Autodesk Inventor part; units mm, degrees
(part 5 of 6)
  arc A2268 (-444.6554, 18.0951) -> (-444.477, 18.6759) centre (-445.0102, 18.5219) ccw
  arc A2269 (-444.477, 18.6759) -> (-444.8927, 19.0646) centre (-445.0103, 18.5222) ccw
  arc A2270 (-444.8927, 19.0646) -> (-445.2136, 19.0814) centre (-445.1047, 18.0874) ccw
  arc A2271 (-445.3689, 19.174) -> (-445.2136, 19.0814) centre (-445.23, 19.2305) ccw
  arc A2272 (-445.5028, 19.7209) -> (-445.3689, 19.174) centre (-421.46, 25.315) ccw
  arc A2273 (-445.4078, 19.8747) -> (-445.5028, 19.7209) centre (-445.3534, 19.7349) ccw
  arc A2274 (-445.4078, 19.8747) -> (-445.1309, 20.0378) centre (-445.7702, 20.8067) ccw
  arc A2275 (-445.1309, 20.0378) -> (-444.9417, 20.5746) centre (-445.4857, 20.4646) ccw
  arc A2276 (-444.9417, 20.5746) -> (-445.3681, 21.0073) centre (-445.4858, 20.4649) ccw
  arc A2277 (-445.3681, 21.0073) -> (-445.6891, 21.0241) centre (-445.5801, 20.03) ccw
  arc A2278 (-445.7718, 21.0387) -> (-445.6891, 21.0241) centre (-445.7054, 21.1732) ccw
  arc A2279 (-445.8827, 21.7261) -> (-445.7718, 21.0387) centre (-421.46, 25.315) ccw
  arc A2280 (-445.8088, 21.7659) -> (-445.8827, 21.7261) centre (-445.7774, 21.6192) ccw
  arc A2281 (-445.8088, 21.7659) -> (-445.5094, 21.8828) centre (-446.0181, 22.7438) ccw
  arc A2282 (-445.5094, 21.8828) -> (-445.2408, 22.4277) centre (-445.7917, 22.3606) ccw
  arc A2283 (-445.2408, 22.4277) -> (-445.5892, 22.8777) centre (-445.7917, 22.361) ccw
  arc A2284 (-445.5892, 22.8777) -> (-445.9034, 22.9454) centre (-445.9542, 21.9467) ccw
  arc A2285 (-446.0419, 23.0615) -> (-445.9034, 22.9454) centre (-445.8958, 23.0952) ccw
  arc A2286 (-446.0869, 23.6228) -> (-446.0419, 23.0615) centre (-421.46, 25.315) ccw
  arc A2287 (-445.9687, 23.7595) -> (-446.0869, 23.6228) centre (-445.9373, 23.6128) ccw
  arc A2288 (-445.9687, 23.7595) -> (-445.6693, 23.8764) centre (-446.1779, 24.7374) ccw
  arc A2289 (-445.6693, 23.8764) -> (-445.397, 24.3762) centre (-445.9516, 24.3542) ccw
  arc A2290 (-445.397, 24.3762) -> (-445.749, 24.8713) centre (-445.9516, 24.3546) ccw
  arc A2291 (-445.749, 24.8713) -> (-446.0632, 24.939) centre (-446.114, 23.9403) ccw
  arc A2292 (-446.1425, 24.9666) -> (-446.0632, 24.939) centre (-446.0556, 25.0888) ccw
  arc A2293 (-446.1425, 25.6629) -> (-446.1425, 24.9666) centre (-421.46, 25.315) ccw
  arc A2294 (-446.0632, 25.6905) -> (-446.1425, 25.6629) centre (-446.0556, 25.5406) ccw
  arc A2295 (-446.0632, 25.6905) -> (-445.749, 25.7581) centre (-446.114, 26.6892) ccw
  arc A2296 (-445.749, 25.7581) -> (-445.397, 26.2533) centre (-445.9516, 26.2749) ccw
  arc A2297 (-445.397, 26.2533) -> (-445.6693, 26.7531) centre (-445.9516, 26.2752) ccw
  arc A2298 (-445.6693, 26.7531) -> (-445.9687, 26.8699) centre (-446.1779, 25.8921) ccw
  arc A2299 (-446.087, 27.0066) -> (-445.9687, 26.8699) centre (-445.9373, 27.0166) ccw
  arc A2300 (-446.042, 27.5679) -> (-446.087, 27.0066) centre (-421.46, 25.315) ccw
  arc A2301 (-445.9034, 27.6841) -> (-446.042, 27.5679) centre (-445.8958, 27.5343) ccw
  arc A2302 (-445.9034, 27.6841) -> (-445.5892, 27.7518) centre (-445.9542, 28.6828) ccw
  arc A2303 (-445.5892, 27.7518) -> (-445.2408, 28.2018) centre (-445.7918, 28.2685) ccw
  arc A2304 (-445.2408, 28.2018) -> (-445.5095, 28.7467) centre (-445.7918, 28.2688) ccw
  arc A2305 (-445.5095, 28.7467) -> (-445.8089, 28.8635) centre (-446.0181, 27.8857) ccw
  arc A2306 (-445.8828, 28.9034) -> (-445.8089, 28.8635) centre (-445.7775, 29.0102) ccw
  arc A2307 (-445.7719, 29.5908) -> (-445.8828, 28.9034) centre (-421.46, 25.315) ccw
  arc A2308 (-445.6892, 29.6054) -> (-445.7719, 29.5908) centre (-445.7055, 29.4563) ccw
  arc A2309 (-445.6892, 29.6054) -> (-445.3682, 29.6222) centre (-445.5802, 30.5994) ccw
  arc A2310 (-445.3682, 29.6222) -> (-444.9418, 30.0549) centre (-445.4859, 30.1646) ccw
  arc A2311 (-444.9418, 30.0549) -> (-445.131, 30.5917) centre (-445.4858, 30.1649) ccw
  arc A2312 (-445.131, 30.5917) -> (-445.4079, 30.7548) centre (-445.7703, 29.8227) ccw
  arc A2313 (-445.5029, 30.9086) -> (-445.4079, 30.7548) centre (-445.3536, 30.8946) ccw
  arc A2314 (-445.3691, 31.4555) -> (-445.5029, 30.9086) centre (-421.46, 25.315) ccw
  arc A2315 (-445.2138, 31.5481) -> (-445.3691, 31.4555) centre (-445.2301, 31.399) ccw
  arc A2316 (-445.2138, 31.5481) -> (-444.8928, 31.5649) centre (-445.1048, 32.5421) ccw
  arc A2317 (-444.8928, 31.5649) -> (-444.4772, 31.9536) centre (-445.0105, 32.1072) ccw
  arc A2318 (-444.4772, 31.9536) -> (-444.6556, 32.5344) centre (-445.0104, 32.1076) ccw
  arc A2319 (-444.6556, 32.5344) -> (-444.9325, 32.6974) centre (-445.2949, 31.7654) ccw
  arc A2320 (-444.9991, 32.7486) -> (-444.9325, 32.6974) centre (-444.8782, 32.8372) ccw
  arc A2321 (-444.7801, 33.4095) -> (-444.9991, 32.7486) centre (-421.46, 25.315) ccw
  arc A2322 (-444.6961, 33.4107) -> (-444.7801, 33.4095) centre (-444.736, 33.2661) ccw
  arc A2323 (-444.6961, 33.4107) -> (-444.3766, 33.3762) centre (-444.4302, 34.3747) ccw
  arc A2324 (-444.3766, 33.3762) -> (-443.8867, 33.7355) centre (-444.4064, 33.9304) ccw
  arc A2325 (-443.8867, 33.7355) -> (-443.988, 34.2955) centre (-444.4062, 33.9307) ccw
  arc A2326 (-443.988, 34.2955) -> (-444.2354, 34.5006) centre (-444.7416, 33.6382) ccw
  arc A2327 (-444.3047, 34.6676) -> (-444.2354, 34.5006) centre (-444.1594, 34.63) ccw
  arc A2328 (-444.0854, 35.1862) -> (-444.3047, 34.6676) centre (-421.46, 25.315) ccw
  arc A2329 (-443.9173, 35.2529) -> (-444.0854, 35.1862) centre (-443.9572, 35.1083) ccw
  arc A2330 (-443.9173, 35.2529) -> (-443.5978, 35.2183) centre (-443.6514, 36.2169) ccw
  arc A2331 (-443.5978, 35.2183) -> (-443.1255, 35.5359) centre (-443.6276, 35.7725) ccw
  arc A2332 (-443.1255, 35.5359) -> (-443.2091, 36.1376) centre (-443.6274, 35.7728) ccw
  arc A2333 (-443.2091, 36.1376) -> (-443.4566, 36.3427) centre (-443.9628, 35.4803) ccw
  arc A2334 (-443.5142, 36.4038) -> (-443.4566, 36.3427) centre (-443.3806, 36.4721) ccw
  arc A2335 (-443.1927, 37.0214) -> (-443.5142, 36.4038) centre (-421.46, 25.315) ccw
  arc A2336 (-443.1096, 37.0093) -> (-443.1927, 37.0214) centre (-443.172, 36.8729) ccw
  arc A2337 (-443.1096, 37.0093) -> (-442.7996, 36.9242) centre (-442.6934, 37.9186) ccw
  arc A2338 (-442.7996, 36.9242) -> (-442.2587, 37.2009) centre (-442.7407, 37.4761) ccw
  arc A2339 (-442.2587, 37.2009) -> (-442.2695, 37.7699) centre (-442.7405, 37.4764) ccw
  arc A2340 (-442.2695, 37.7699) -> (-442.481, 38.0118) centre (-443.1182, 37.2411) ccw
  arc A2341 (-442.5228, 38.1877) -> (-442.481, 38.0118) centre (-442.3855, 38.1274) ccw
  arc A2342 (-442.2237, 38.6648) -> (-442.5228, 38.1877) centre (-421.46, 25.315) ccw
  arc A2343 (-442.0472, 38.7038) -> (-442.2237, 38.6648) centre (-442.1096, 38.5674) ccw
  arc A2344 (-442.0472, 38.7038) -> (-441.7373, 38.6188) centre (-441.6311, 39.6131) ccw
  arc A2345 (-441.7373, 38.6188) -> (-441.2204, 38.857) centre (-441.6783, 39.1706) ccw
  arc A2346 (-441.2204, 38.857) -> (-441.2071, 39.4644) centre (-441.6781, 39.1709) ccw
  arc A2347 (-441.2071, 39.4644) -> (-441.4187, 39.7063) centre (-442.0558, 38.9356) ccw
  arc A2348 (-441.4658, 39.7758) -> (-441.4187, 39.7063) centre (-441.3231, 39.822) ccw
  arc A2349 (-441.05, 40.3343) -> (-441.4658, 39.7758) centre (-421.46, 25.315) ccw
  arc A2350 (-440.9699, 40.3091) -> (-441.05, 40.3343) centre (-441.0533, 40.1844) ccw
  arc A2351 (-440.9699, 40.3091) -> (-440.6775, 40.1757) centre (-440.4142, 41.1405) ccw
  arc A2352 (-440.6775, 40.1757) -> (-440.0994, 40.3627) centre (-440.5314, 40.7112) ccw
  arc A2353 (-440.0994, 40.3627) -> (-440.0194, 40.9262) centre (-440.5312, 40.7115) ccw
  arc A2354 (-440.0194, 40.9262) -> (-440.1897, 41.1987) centre (-440.9415, 40.5393) ccw
  arc A2355 (-440.2029, 41.379) -> (-440.1897, 41.1987) centre (-440.0769, 41.2976) ccw
  arc A2356 (-439.8317, 41.8023) -> (-440.2029, 41.379) centre (-421.46, 25.315) ccw
  arc A2357 (-439.6512, 41.8127) -> (-439.8317, 41.8023) centre (-439.7345, 41.688) ccw
  arc A2358 (-439.6512, 41.8127) -> (-439.3587, 41.6794) centre (-439.0955, 42.6441) ccw
  arc A2359 (-439.3587, 41.6794) -> (-438.8105, 41.8323) centre (-439.2126, 42.2148) ccw
  arc A2360 (-438.8105, 41.8323) -> (-438.7006, 42.4298) centre (-439.2124, 42.2151) ccw
  arc A2361 (-438.7006, 42.4298) -> (-438.8709, 42.7023) centre (-439.6228, 42.0429) ccw
  arc A2362 (-438.9064, 42.7784) -> (-438.8709, 42.7023) centre (-438.7582, 42.8012) ccw
  arc A2363 (-438.4069, 43.2635) -> (-438.9064, 42.7784) centre (-421.46, 25.315) ccw
  arc A2364 (-438.3319, 43.2258) -> (-438.4069, 43.2635) centre (-438.4341, 43.116) ccw
  arc A2365 (-438.3319, 43.2258) -> (-438.0644, 43.0476) centre (-437.6509, 43.9581) ccw
  arc A2366 (-438.0644, 43.0476) -> (-437.464, 43.1401) centre (-437.8349, 43.5529) ccw
  arc A2367 (-437.464, 43.1401) -> (-437.2952, 43.6836) centre (-437.8346, 43.5532) ccw
  arc A2368 (-437.2952, 43.6836) -> (-437.4199, 43.9798) centre (-438.2672, 43.4486) ccw
  arc A2369 (-437.4043, 44.1599) -> (-437.4199, 43.9798) centre (-437.2928, 44.0595) ccw
  arc A2370 (-436.9703, 44.5187) -> (-437.4043, 44.1599) centre (-421.46, 25.315) ccw
  arc A2371 (-436.7904, 44.5002) -> (-436.9703, 44.5187) centre (-436.8926, 44.3903) ccw
  arc A2372 (-436.7904, 44.5002) -> (-436.523, 44.322) centre (-436.1094, 45.2324) ccw
  arc A2373 (-436.523, 44.322) -> (-435.9574, 44.3856) centre (-436.2935, 44.8273) ccw
  arc A2374 (-435.9574, 44.3856) -> (-435.7537, 44.9579) centre (-436.2932, 44.8275) ccw
  arc A2375 (-435.7537, 44.9579) -> (-435.8784, 45.2541) centre (-436.7257, 44.7229) ccw
  arc A2376 (-435.9014, 45.3349) -> (-435.8784, 45.2541) centre (-435.7514, 45.3338) ccw
  arc A2377 (-435.331, 45.7342) -> (-435.9014, 45.3349) centre (-421.46, 25.315) ccw
  arc A2378 (-435.2629, 45.6851) -> (-435.331, 45.7342) centre (-435.3812, 45.5929) ccw
  arc A2379 (-435.2629, 45.6851) -> (-435.0272, 45.4665) centre (-434.4739, 46.2995) ccw
  arc A2380 (-435.0272, 45.4665) -> (-434.4197, 45.4621) centre (-434.7201, 45.9288) ccw
  arc A2381 (-434.4197, 45.4621) -> (-434.1665, 45.9718) centre (-434.7198, 45.929) ccw
  arc A2382 (-434.1665, 45.9718) -> (-434.2424, 46.2841) centre (-435.1635, 45.8947) ccw
  arc A2383 (-434.1983, 46.4594) -> (-434.2424, 46.2841) centre (-434.1043, 46.3425) ccw
  arc A2384 (-433.7127, 46.7445) -> (-434.1983, 46.4594) centre (-421.46, 25.315) ccw
  arc A2385 (-433.5381, 46.6976) -> (-433.7127, 46.7445) centre (-433.6564, 46.6054) ccw
  arc A2386 (-433.5381, 46.6976) -> (-433.3024, 46.479) centre (-432.7491, 47.3119) ccw
  arc A2387 (-433.3024, 46.479) -> (-432.734, 46.4517) centre (-432.9953, 46.9413) ccw
  arc A2388 (-432.734, 46.4517) -> (-432.4417, 46.9843) centre (-432.995, 46.9415) ccw
  arc A2389 (-432.4417, 46.9843) -> (-432.5176, 47.2965) centre (-433.4387, 46.9071) ccw
  arc A2390 (-432.5274, 47.38) -> (-432.5176, 47.2965) centre (-432.3795, 47.355) ccw
  arc A2391 (-431.9006, 47.6833) -> (-432.5274, 47.38) centre (-421.46, 25.315) ccw
  arc A2392 (-431.8412, 47.6239) -> (-431.9006, 47.6833) centre (-431.9728, 47.5518) ccw
  arc A2393 (-431.8412, 47.6239) -> (-431.6434, 47.3706) centre (-430.9644, 48.1048) ccw
  arc A2394 (-431.6434, 47.3706) -> (-431.0444, 47.2695) centre (-431.2666, 47.7781) ccw
  arc A2395 (-431.0444, 47.2695) -> (-430.7132, 47.7323) centre (-431.2663, 47.7782) ccw
  arc A2396 (-430.7132, 47.7323) -> (-430.7384, 48.0527) centre (-431.7097, 47.815) ccw
  arc A2397 (-430.6669, 48.2188) -> (-430.7384, 48.0527) centre (-430.5927, 48.0884) ccw
  arc A2398 (-430.1421, 48.4228) -> (-430.6669, 48.2188) centre (-421.46, 25.315) ccw
  arc A2399 (-429.9772, 48.3487) -> (-430.1421, 48.4228) centre (-430.1087, 48.2766) ccw
  arc A2400 (-429.9772, 48.3487) -> (-429.7794, 48.0954) centre (-429.1004, 48.8295) ccw
  arc A2401 (-429.7794, 48.0954) -> (-429.2225, 47.9779) centre (-429.4025, 48.5028) ccw
  arc A2402 (-429.2225, 47.9779) -> (-428.8491, 48.4571) centre (-429.4022, 48.503) ccw
  arc A2403 (-428.8491, 48.4571) -> (-428.8743, 48.7775) centre (-429.8457, 48.5398) ccw
  arc A2404 (-428.8707, 48.8614) -> (-428.8743, 48.7775) centre (-428.7286, 48.8131) ccw
  arc A2405 (-428.2036, 49.061) -> (-428.8707, 48.8614) centre (-421.46, 25.315) ccw
  arc A2406 (-428.1544, 48.9929) -> (-428.2036, 49.061) centre (-428.2958, 48.9427) ccw
  arc A2407 (-428.1544, 48.9929) -> (-427.9995, 48.7113) centre (-427.2122, 49.3279) ccw
  arc A2408 (-427.9995, 48.7113) -> (-427.4242, 48.5161) centre (-427.5626, 49.0536) ccw
  arc A2409 (-427.4242, 48.5161) -> (-427.0235, 48.9202) centre (-427.5622, 49.0536) ccw
  arc A2410 (-427.0235, 48.9202) -> (-426.9974, 49.2405) centre (-427.9942, 49.1606) ccw
  arc A2411 (-426.9003, 49.393) -> (-426.9974, 49.2405) centre (-426.8478, 49.2525) ccw
  arc A2412 (-426.3497, 49.5109) -> (-426.9003, 49.393) centre (-421.46, 25.315) ccw
  arc A2413 (-426.1987, 49.4114) -> (-426.3497, 49.5109) centre (-426.34, 49.3612) ccw
  arc A2414 (-426.1987, 49.4114) -> (-426.0438, 49.1299) centre (-425.2565, 49.7465) ccw
  arc A2415 (-426.0438, 49.1299) -> (-425.5128, 48.9251) centre (-425.6068, 49.4721) ccw
  arc A2416 (-425.5128, 48.9251) -> (-425.0678, 49.3387) centre (-425.6065, 49.4721) ccw
  arc A2417 (-425.0678, 49.3387) -> (-425.0416, 49.659) centre (-426.0384, 49.5791) ccw
  arc A2418 (-425.0246, 49.7413) -> (-425.0416, 49.659) centre (-424.8921, 49.671) ccw
  arc A2419 (-424.3343, 49.8321) -> (-425.0246, 49.7413) centre (-421.46, 25.315) ccw
  arc A2420 (-424.2966, 49.757) -> (-424.3343, 49.8321) centre (-424.4441, 49.7299) ccw
  arc A2421 (-424.2966, 49.757) -> (-424.1885, 49.4544) centre (-423.313, 49.9377) ccw
  arc A2422 (-424.1885, 49.4544) -> (-423.6517, 49.1699) centre (-423.7026, 49.7226) ccw
  arc A2423 (-423.6517, 49.1699) -> (-423.1917, 49.5051) centre (-423.7023, 49.7226) ccw
  arc A2424 (-423.1917, 49.5051) -> (-423.1149, 49.8171) centre (-424.1117, 49.8971) ccw
  arc A2425 (-422.9947, 49.9522) -> (-423.1149, 49.8171) centre (-422.9653, 49.8052) ccw
  arc A2426 (-422.4324, 49.9808) -> (-422.9947, 49.9522) centre (-421.46, 25.315) ccw
  arc A2427 (-422.2992, 49.8586) -> (-422.4324, 49.9808) centre (-422.4467, 49.8315) ccw
  arc A2428 (-422.2992, 49.8586) -> (-422.1911, 49.556) centre (-421.3156, 50.0392) ccw
  arc A2429 (-422.1911, 49.556) -> (-421.6995, 49.2692) centre (-421.7052, 49.8242) ccw
  arc A2430 (-421.6995, 49.2692) -> (-421.1943, 49.6066) centre (-421.7048, 49.8242) ccw
  arc A2431 (-421.1943, 49.6066) -> (-421.1174, 49.9187) centre (-422.1142, 49.9986) ccw
  arc A2432 (-421.0854, 50) -> (-421.1174, 49.9187) centre (-420.9679, 49.9067) ccw
  line L316 (-421.0854, 50) -> (-420.4705, 50)
  arc A2433 (-420.3218, 49.8696) -> (-420.4705, 50) centre (-420.4705, 49.85) ccw
  arc A2434 (-420.3218, 49.8696) -> (-420.2292, 49.5618) centre (-419.3304, 50) ccw
  arc A2435 (-420.2292, 49.5618) -> (-419.7302, 49.25) centre (-419.7304, 49.805) ccw
  arc A2436 (-419.7302, 49.25) -> (-419.2311, 49.5618) centre (-419.73, 49.805) ccw
  arc A2437 (-419.2311, 49.5618) -> (-419.1385, 49.8696) centre (-420.13, 50) ccw
  arc A2438 (-418.9898, 50) -> (-419.1385, 49.8696) centre (-418.9898, 49.85) ccw
  line L317 (-418.9898, 50) -> (-418.4705, 50)
  arc A2439 (-418.3218, 49.8696) -> (-418.4705, 50) centre (-418.4705, 49.85) ccw
  arc A2440 (-418.3218, 49.8696) -> (-418.2292, 49.5618) centre (-417.3304, 50) ccw
  arc A2441 (-418.2292, 49.5618) -> (-417.7302, 49.25) centre (-417.7304, 49.805) ccw
  arc A2442 (-417.7302, 49.25) -> (-417.2311, 49.5618) centre (-417.73, 49.805) ccw
  arc A2443 (-417.2311, 49.5618) -> (-417.1385, 49.8696) centre (-418.13, 50) ccw
  arc A2444 (-416.9898, 50) -> (-417.1385, 49.8696) centre (-416.9898, 49.85) ccw
  line L318 (-416.9898, 50) -> (-416.4705, 50)
  arc A2445 (-416.3218, 49.8696) -> (-416.4705, 50) centre (-416.4705, 49.85) ccw
  arc A2446 (-416.3218, 49.8696) -> (-416.2292, 49.5618) centre (-415.3304, 50) ccw
  arc A2447 (-416.2292, 49.5618) -> (-415.7302, 49.25) centre (-415.7304, 49.805) ccw
  arc A2448 (-415.7302, 49.25) -> (-415.2311, 49.5618) centre (-415.73, 49.805) ccw
  arc A2449 (-415.2311, 49.5618) -> (-415.1385, 49.8696) centre (-416.13, 50) ccw
  arc A2450 (-414.9898, 50) -> (-415.1385, 49.8696) centre (-414.9898, 49.85) ccw
  line L319 (-414.9898, 50) -> (-414.4705, 50)
  arc A2451 (-414.3218, 49.8696) -> (-414.4705, 50) centre (-414.4705, 49.85) ccw
  arc A2452 (-414.3218, 49.8696) -> (-414.2292, 49.5618) centre (-413.3304, 50) ccw
  arc A2453 (-414.2292, 49.5618) -> (-413.7302, 49.25) centre (-413.7304, 49.805) ccw
  arc A2454 (-413.7302, 49.25) -> (-413.2311, 49.5618) centre (-413.73, 49.805) ccw
  arc A2455 (-413.2311, 49.5618) -> (-413.1385, 49.8696) centre (-414.13, 50) ccw
  arc A2456 (-412.9898, 50) -> (-413.1385, 49.8696) centre (-412.9898, 49.85) ccw
  line L320 (-412.9898, 50) -> (-412.4705, 50)
  arc A2457 (-412.3218, 49.8696) -> (-412.4705, 50) centre (-412.4705, 49.85) ccw
  arc A2458 (-412.3218, 49.8696) -> (-412.2292, 49.5618) centre (-411.3304, 50) ccw
  arc A2459 (-412.2292, 49.5618) -> (-411.7302, 49.25) centre (-411.7304, 49.805) ccw
  arc A2460 (-411.7302, 49.25) -> (-411.2311, 49.5618) centre (-411.73, 49.805) ccw
  arc A2461 (-411.2311, 49.5618) -> (-411.1385, 49.8696) centre (-412.13, 50) ccw
  arc A2462 (-410.9898, 50) -> (-411.1385, 49.8696) centre (-410.9898, 49.85) ccw
  line L321 (-410.9898, 50) -> (-410.4705, 50)
  arc A2463 (-410.3218, 49.8696) -> (-410.4705, 50) centre (-410.4705, 49.85) ccw
  arc A2464 (-410.3218, 49.8696) -> (-410.2292, 49.5618) centre (-409.3304, 50) ccw
  arc A2465 (-410.2292, 49.5618) -> (-409.7302, 49.25) centre (-409.7304, 49.805) ccw
  arc A2466 (-409.7302, 49.25) -> (-409.2311, 49.5618) centre (-409.73, 49.805) ccw
  arc A2467 (-409.2311, 49.5618) -> (-409.1385, 49.8696) centre (-410.13, 50) ccw
  arc A2468 (-408.9898, 50) -> (-409.1385, 49.8696) centre (-408.9898, 49.85) ccw
  line L322 (-408.9898, 50) -> (-408.4705, 50)
  arc A2469 (-408.3218, 49.8696) -> (-408.4705, 50) centre (-408.4705, 49.85) ccw
  arc A2470 (-408.3218, 49.8696) -> (-408.2292, 49.5618) centre (-407.3304, 50) ccw
  arc A2471 (-408.2292, 49.5618) -> (-407.7302, 49.25) centre (-407.7304, 49.805) ccw
  arc A2472 (-407.7302, 49.25) -> (-407.2311, 49.5618) centre (-407.73, 49.805) ccw
  arc A2473 (-407.2311, 49.5618) -> (-407.1385, 49.8696) centre (-408.13, 50) ccw
  arc A2474 (-406.9898, 50) -> (-407.1385, 49.8696) centre (-406.9898, 49.85) ccw
  line L323 (-406.9898, 50) -> (-406.4705, 50)
  arc A2475 (-406.3218, 49.8696) -> (-406.4705, 50) centre (-406.4705, 49.85) ccw
  arc A2476 (-406.3218, 49.8696) -> (-406.2292, 49.5618) centre (-405.3304, 50) ccw
  arc A2477 (-406.2292, 49.5618) -> (-405.7302, 49.25) centre (-405.7304, 49.805) ccw
  arc A2478 (-405.7302, 49.25) -> (-405.2311, 49.5618) centre (-405.73, 49.805) ccw
  arc A2479 (-405.2311, 49.5618) -> (-405.1385, 49.8696) centre (-406.13, 50) ccw
  arc A2480 (-404.9898, 50) -> (-405.1385, 49.8696) centre (-404.9898, 49.85) ccw
  line L324 (-404.9898, 50) -> (-404.4705, 50)
  arc A2481 (-404.3218, 49.8696) -> (-404.4705, 50) centre (-404.4705, 49.85) ccw
  arc A2482 (-404.3218, 49.8696) -> (-404.2292, 49.5618) centre (-403.3304, 50) ccw
  arc A2483 (-404.2292, 49.5618) -> (-403.7302, 49.25) centre (-403.7304, 49.805) ccw
  arc A2484 (-403.7302, 49.25) -> (-403.2311, 49.5618) centre (-403.73, 49.805) ccw
  arc A2485 (-403.2311, 49.5618) -> (-403.1385, 49.8696) centre (-404.13, 50) ccw
  arc A2486 (-402.9898, 50) -> (-403.1385, 49.8696) centre (-402.9898, 49.85) ccw
  line L325 (-402.9898, 50) -> (-402.4705, 50)
  arc A2487 (-402.3218, 49.8696) -> (-402.4705, 50) centre (-402.4705, 49.85) ccw
  arc A2488 (-402.3218, 49.8696) -> (-402.2292, 49.5618) centre (-401.3304, 50) ccw
  arc A2489 (-402.2292, 49.5618) -> (-401.7302, 49.25) centre (-401.7304, 49.805) ccw
  arc A2490 (-401.7302, 49.25) -> (-401.2311, 49.5618) centre (-401.73, 49.805) ccw
  arc A2491 (-401.2311, 49.5618) -> (-401.1385, 49.8696) centre (-402.13, 50) ccw
  arc A2492 (-400.9898, 50) -> (-401.1385, 49.8696) centre (-400.9898, 49.85) ccw
  line L326 (-400.9898, 50) -> (-400.4705, 50)
  arc A2493 (-400.3218, 49.8696) -> (-400.4705, 50) centre (-400.4705, 49.85) ccw
  arc A2494 (-400.3218, 49.8696) -> (-400.2292, 49.5618) centre (-399.3304, 50) ccw
  arc A2495 (-400.2292, 49.5618) -> (-399.7302, 49.25) centre (-399.7304, 49.805) ccw
  arc A2496 (-399.7302, 49.25) -> (-399.2311, 49.5618) centre (-399.73, 49.805) ccw
  arc A2497 (-399.2311, 49.5618) -> (-399.1385, 49.8696) centre (-400.13, 50) ccw
  arc A2498 (-398.9898, 50) -> (-399.1385, 49.8696) centre (-398.9898, 49.85) ccw
  line L327 (-398.9898, 50) -> (-398.4705, 50)
  arc A2499 (-398.3218, 49.8696) -> (-398.4705, 50) centre (-398.4705, 49.85) ccw
  arc A2500 (-398.3218, 49.8696) -> (-398.2292, 49.5618) centre (-397.3304, 50) ccw
  arc A2501 (-398.2292, 49.5618) -> (-397.7302, 49.25) centre (-397.7304, 49.805) ccw
  arc A2502 (-397.7302, 49.25) -> (-397.2311, 49.5618) centre (-397.73, 49.805) ccw
  arc A2503 (-397.2311, 49.5618) -> (-397.1385, 49.8696) centre (-398.13, 50) ccw
  arc A2504 (-396.9898, 50) -> (-397.1385, 49.8696) centre (-396.9898, 49.85) ccw
  line L328 (-396.9898, 50) -> (-396.4705, 50)
  arc A2505 (-396.3218, 49.8696) -> (-396.4705, 50) centre (-396.4705, 49.85) ccw
  arc A2506 (-396.3218, 49.8696) -> (-396.2292, 49.5618) centre (-395.3304, 50) ccw
  arc A2507 (-396.2292, 49.5618) -> (-395.7302, 49.25) centre (-395.7304, 49.805) ccw
  arc A2508 (-395.7302, 49.25) -> (-395.2311, 49.5618) centre (-395.73, 49.805) ccw
  arc A2509 (-395.2311, 49.5618) -> (-395.1385, 49.8696) centre (-396.13, 50) ccw
  arc A2510 (-394.9898, 50) -> (-395.1385, 49.8696) centre (-394.9898, 49.85) ccw
  line L329 (-394.9898, 50) -> (-394.4705, 50)
  arc A2511 (-394.3218, 49.8696) -> (-394.4705, 50) centre (-394.4705, 49.85) ccw
  arc A2512 (-394.3218, 49.8696) -> (-394.2292, 49.5618) centre (-393.3304, 50) ccw
  arc A2513 (-394.2292, 49.5618) -> (-393.7302, 49.25) centre (-393.7304, 49.805) ccw
  arc A2514 (-393.7302, 49.25) -> (-393.2311, 49.5618) centre (-393.73, 49.805) ccw
  arc A2515 (-393.2311, 49.5618) -> (-393.1385, 49.8696) centre (-394.13, 50) ccw
  arc A2516 (-392.9898, 50) -> (-393.1385, 49.8696) centre (-392.9898, 49.85) ccw
  line L330 (-392.9898, 50) -> (-392.4705, 50)
  arc A2517 (-392.3218, 49.8696) -> (-392.4705, 50) centre (-392.4705, 49.85) ccw
  arc A2518 (-392.3218, 49.8696) -> (-392.2292, 49.5618) centre (-391.3304, 50) ccw
  arc A2519 (-392.2292, 49.5618) -> (-391.7302, 49.25) centre (-391.7304, 49.805) ccw
  arc A2520 (-391.7302, 49.25) -> (-391.2311, 49.5618) centre (-391.73, 49.805) ccw
  arc A2521 (-391.2311, 49.5618) -> (-391.1385, 49.8696) centre (-392.13, 50) ccw
  arc A2522 (-390.9898, 50) -> (-391.1385, 49.8696) centre (-390.9898, 49.85) ccw
  line L331 (-390.9898, 50) -> (-390.4705, 50)
  arc A2523 (-390.3218, 49.8696) -> (-390.4705, 50) centre (-390.4705, 49.85) ccw
  arc A2524 (-390.3218, 49.8696) -> (-390.2292, 49.5618) centre (-389.3304, 50) ccw
  arc A2525 (-390.2292, 49.5618) -> (-389.7302, 49.25) centre (-389.7304, 49.805) ccw
  arc A2526 (-389.7302, 49.25) -> (-389.2311, 49.5618) centre (-389.73, 49.805) ccw
  arc A2527 (-389.2311, 49.5618) -> (-389.1385, 49.8696) centre (-390.13, 50) ccw
  arc A2528 (-388.9898, 50) -> (-389.1385, 49.8696) centre (-388.9898, 49.85) ccw
  line L332 (-388.9898, 50) -> (-388.4705, 50)
  arc A2529 (-388.3218, 49.8696) -> (-388.4705, 50) centre (-388.4705, 49.85) ccw
  arc A2530 (-388.3218, 49.8696) -> (-388.2292, 49.5618) centre (-387.3304, 50) ccw
  arc A2531 (-388.2292, 49.5618) -> (-387.7302, 49.25) centre (-387.7304, 49.805) ccw
  arc A2532 (-387.7302, 49.25) -> (-387.2311, 49.5618) centre (-387.73, 49.805) ccw
  arc A2533 (-387.2311, 49.5618) -> (-387.1385, 49.8696) centre (-388.13, 50) ccw
  arc A2534 (-386.9898, 50) -> (-387.1385, 49.8696) centre (-386.9898, 49.85) ccw
  line L333 (-386.9898, 50) -> (-386.4705, 50)
  arc A2535 (-386.3218, 49.8696) -> (-386.4705, 50) centre (-386.4705, 49.85) ccw
  arc A2536 (-386.3218, 49.8696) -> (-386.2292, 49.5618) centre (-385.3304, 50) ccw
  arc A2537 (-386.2292, 49.5618) -> (-385.7302, 49.25) centre (-385.7304, 49.805) ccw
  arc A2538 (-385.7302, 49.25) -> (-385.2311, 49.5618) centre (-385.73, 49.805) ccw
  arc A2539 (-385.2311, 49.5618) -> (-385.1385, 49.8696) centre (-386.13, 50) ccw
  arc A2540 (-384.9898, 50) -> (-385.1385, 49.8696) centre (-384.9898, 49.85) ccw
  line L334 (-384.9898, 50) -> (-384.4705, 50)
  arc A2541 (-384.3218, 49.8696) -> (-384.4705, 50) centre (-384.4705, 49.85) ccw
  arc A2542 (-384.3218, 49.8696) -> (-384.2292, 49.5618) centre (-383.3304, 50) ccw
  arc A2543 (-384.2292, 49.5618) -> (-383.7302, 49.25) centre (-383.7304, 49.805) ccw
  arc A2544 (-383.7302, 49.25) -> (-383.2311, 49.5618) centre (-383.73, 49.805) ccw
  arc A2545 (-383.2311, 49.5618) -> (-383.1385, 49.8696) centre (-384.13, 50) ccw
  arc A2546 (-382.9898, 50) -> (-383.1385, 49.8696) centre (-382.9898, 49.85) ccw
  line L335 (-382.9898, 50) -> (-382.4705, 50)
  arc A2547 (-382.3218, 49.8696) -> (-382.4705, 50) centre (-382.4705, 49.85) ccw
  arc A2548 (-382.3218, 49.8696) -> (-382.2292, 49.5618) centre (-381.3304, 50) ccw
  arc A2549 (-382.2292, 49.5618) -> (-381.7302, 49.25) centre (-381.7304, 49.805) ccw
  arc A2550 (-381.7302, 49.25) -> (-381.2311, 49.5618) centre (-381.73, 49.805) ccw
  arc A2551 (-381.2311, 49.5618) -> (-381.1385, 49.8696) centre (-382.13, 50) ccw
  arc A2552 (-380.9898, 50) -> (-381.1385, 49.8696) centre (-380.9898, 49.85) ccw
  line L336 (-380.9898, 50) -> (-380.4705, 50)
  arc A2553 (-380.3218, 49.8696) -> (-380.4705, 50) centre (-380.4705, 49.85) ccw
  arc A2554 (-380.3218, 49.8696) -> (-380.2292, 49.5618) centre (-379.3304, 50) ccw
  arc A2555 (-380.2292, 49.5618) -> (-379.7302, 49.25) centre (-379.7304, 49.805) ccw
  arc A2556 (-379.7302, 49.25) -> (-379.2311, 49.5618) centre (-379.73, 49.805) ccw
  arc A2557 (-379.2311, 49.5618) -> (-379.1385, 49.8696) centre (-380.13, 50) ccw
  arc A2558 (-378.9898, 50) -> (-379.1385, 49.8696) centre (-378.9898, 49.85) ccw
  line L337 (-378.9898, 50) -> (-378.4705, 50)
  arc A2559 (-378.3218, 49.8696) -> (-378.4705, 50) centre (-378.4705, 49.85) ccw
  arc A2560 (-378.3218, 49.8696) -> (-378.2292, 49.5618) centre (-377.3304, 50) ccw
  arc A2561 (-378.2292, 49.5618) -> (-377.7302, 49.25) centre (-377.7304, 49.805) ccw
  arc A2562 (-377.7302, 49.25) -> (-377.2311, 49.5618) centre (-377.73, 49.805) ccw
  arc A2563 (-377.2311, 49.5618) -> (-377.1385, 49.8696) centre (-378.13, 50) ccw
  arc A2564 (-376.9898, 50) -> (-377.1385, 49.8696) centre (-376.9898, 49.85) ccw
  line L338 (-376.9898, 50) -> (-376.4705, 50)
  arc A2565 (-376.3218, 49.8696) -> (-376.4705, 50) centre (-376.4705, 49.85) ccw
  arc A2566 (-376.3218, 49.8696) -> (-376.2292, 49.5618) centre (-375.3304, 50) ccw
  arc A2567 (-376.2292, 49.5618) -> (-375.7302, 49.25) centre (-375.7304, 49.805) ccw
  arc A2568 (-375.7302, 49.25) -> (-375.2311, 49.5618) centre (-375.73, 49.805) ccw
  arc A2569 (-375.2311, 49.5618) -> (-375.1385, 49.8696) centre (-376.13, 50) ccw
  arc A2570 (-374.9898, 50) -> (-375.1385, 49.8696) centre (-374.9898, 49.85) ccw
  line L339 (-374.9898, 50) -> (-374.4705, 50)
  arc A2571 (-374.3218, 49.8696) -> (-374.4705, 50) centre (-374.4705, 49.85) ccw
  arc A2572 (-374.3218, 49.8696) -> (-374.2292, 49.5618) centre (-373.3304, 50) ccw
  arc A2573 (-374.2292, 49.5618) -> (-373.7302, 49.25) centre (-373.7304, 49.805) ccw
  arc A2574 (-373.7302, 49.25) -> (-373.2311, 49.5618) centre (-373.73, 49.805) ccw
  arc A2575 (-373.2311, 49.5618) -> (-373.1385, 49.8696) centre (-374.13, 50) ccw
  arc A2576 (-372.9898, 50) -> (-373.1385, 49.8696) centre (-372.9898, 49.85) ccw
  line L340 (-372.9898, 50) -> (-372.4705, 50)
  arc A2577 (-372.3218, 49.8696) -> (-372.4705, 50) centre (-372.4705, 49.85) ccw
  arc A2578 (-372.3218, 49.8696) -> (-372.2292, 49.5618) centre (-371.3304, 50) ccw
  arc A2579 (-372.2292, 49.5618) -> (-371.7302, 49.25) centre (-371.7304, 49.805) ccw
  arc A2580 (-371.7302, 49.25) -> (-371.2311, 49.5618) centre (-371.73, 49.805) ccw
  arc A2581 (-371.2311, 49.5618) -> (-371.1385, 49.8696) centre (-372.13, 50) ccw
  arc A2582 (-370.9898, 50) -> (-371.1385, 49.8696) centre (-370.9898, 49.85) ccw
  line L341 (-370.9898, 50) -> (-370.4705, 50)
  arc A2583 (-370.3218, 49.8696) -> (-370.4705, 50) centre (-370.4705, 49.85) ccw
  arc A2584 (-370.3218, 49.8696) -> (-370.2292, 49.5618) centre (-369.3304, 50) ccw
  arc A2585 (-370.2292, 49.5618) -> (-369.7302, 49.25) centre (-369.7304, 49.805) ccw
  arc A2586 (-369.7302, 49.25) -> (-369.2311, 49.5618) centre (-369.73, 49.805) ccw
  arc A2587 (-369.2311, 49.5618) -> (-369.1385, 49.8696) centre (-370.13, 50) ccw
  arc A2588 (-368.9898, 50) -> (-369.1385, 49.8696) centre (-368.9898, 49.85) ccw
  line L342 (-368.9898, 50) -> (-368.4705, 50)
  arc A2589 (-368.3218, 49.8696) -> (-368.4705, 50) centre (-368.4705, 49.85) ccw
  arc A2590 (-368.3218, 49.8696) -> (-368.2292, 49.5618) centre (-367.3304, 50) ccw
  arc A2591 (-368.2292, 49.5618) -> (-367.7302, 49.25) centre (-367.7304, 49.805) ccw
  arc A2592 (-367.7302, 49.25) -> (-367.2311, 49.5618) centre (-367.73, 49.805) ccw
  arc A2593 (-367.2311, 49.5618) -> (-367.1385, 49.8696) centre (-368.13, 50) ccw
  arc A2594 (-366.9898, 50) -> (-367.1385, 49.8696) centre (-366.9898, 49.85) ccw
  line L343 (-366.9898, 50) -> (-366.4705, 50)
  arc A2595 (-366.3218, 49.8696) -> (-366.4705, 50) centre (-366.4705, 49.85) ccw
  arc A2596 (-366.3218, 49.8696) -> (-366.2292, 49.5618) centre (-365.3304, 50) ccw
  arc A2597 (-366.2292, 49.5618) -> (-365.7302, 49.25) centre (-365.7304, 49.805) ccw
  arc A2598 (-365.7302, 49.25) -> (-365.2311, 49.5618) centre (-365.73, 49.805) ccw
  arc A2599 (-365.2311, 49.5618) -> (-365.1385, 49.8696) centre (-366.13, 50) ccw
  arc A2600 (-364.9898, 50) -> (-365.1385, 49.8696) centre (-364.9898, 49.85) ccw
  line L344 (-364.9898, 50) -> (-364.4705, 50)
  arc A2601 (-364.3218, 49.8696) -> (-364.4705, 50) centre (-364.4705, 49.85) ccw
  arc A2602 (-364.3218, 49.8696) -> (-364.2292, 49.5618) centre (-363.3304, 50) ccw
  arc A2603 (-364.2292, 49.5618) -> (-363.7302, 49.25) centre (-363.7304, 49.805) ccw
  arc A2604 (-363.7302, 49.25) -> (-363.2311, 49.5618) centre (-363.73, 49.805) ccw
  arc A2605 (-363.2311, 49.5618) -> (-363.1385, 49.8696) centre (-364.13, 50) ccw
  arc A2606 (-362.9898, 50) -> (-363.1385, 49.8696) centre (-362.9898, 49.85) ccw
  line L345 (-362.9898, 50) -> (-362.4705, 50)
  arc A2607 (-362.3218, 49.8696) -> (-362.4705, 50) centre (-362.4705, 49.85) ccw
  arc A2608 (-362.3218, 49.8696) -> (-362.2292, 49.5618) centre (-361.3304, 50) ccw
  arc A2609 (-362.2292, 49.5618) -> (-361.7302, 49.25) centre (-361.7304, 49.805) ccw
  arc A2610 (-361.7302, 49.25) -> (-361.2311, 49.5618) centre (-361.73, 49.805) ccw
  arc A2611 (-361.2311, 49.5618) -> (-361.1385, 49.8696) centre (-362.13, 50) ccw
  arc A2612 (-360.9898, 50) -> (-361.1385, 49.8696) centre (-360.9898, 49.85) ccw
  line L346 (-360.9898, 50) -> (-360.4705, 50)
  arc A2613 (-360.3218, 49.8696) -> (-360.4705, 50) centre (-360.4705, 49.85) ccw
  arc A2614 (-360.3218, 49.8696) -> (-360.2292, 49.5618) centre (-359.3304, 50) ccw
  arc A2615 (-360.2292, 49.5618) -> (-359.7302, 49.25) centre (-359.7304, 49.805) ccw
  arc A2616 (-359.7302, 49.25) -> (-359.2311, 49.5618) centre (-359.73, 49.805) ccw
  arc A2617 (-359.2311, 49.5618) -> (-359.1385, 49.8696) centre (-360.13, 50) ccw
  arc A2618 (-358.9898, 50) -> (-359.1385, 49.8696) centre (-358.9898, 49.85) ccw
  line L347 (-358.9898, 50) -> (-358.4705, 50)
  arc A2619 (-358.3218, 49.8696) -> (-358.4705, 50) centre (-358.4705, 49.85) ccw
  arc A2620 (-358.3218, 49.8696) -> (-358.2292, 49.5618) centre (-357.3304, 50) ccw
  arc A2621 (-358.2292, 49.5618) -> (-357.7302, 49.25) centre (-357.7304, 49.805) ccw
  arc A2622 (-357.7302, 49.25) -> (-357.2311, 49.5618) centre (-357.73, 49.805) ccw
  arc A2623 (-357.2311, 49.5618) -> (-357.1385, 49.8696) centre (-358.13, 50) ccw
  arc A2624 (-356.9898, 50) -> (-357.1385, 49.8696) centre (-356.9898, 49.85) ccw
  line L348 (-356.9898, 50) -> (-356.4705, 50)
  arc A2625 (-356.3218, 49.8696) -> (-356.4705, 50) centre (-356.4705, 49.85) ccw
  arc A2626 (-356.3218, 49.8696) -> (-356.2292, 49.5618) centre (-355.3304, 50) ccw
  arc A2627 (-356.2292, 49.5618) -> (-355.7302, 49.25) centre (-355.7304, 49.805) ccw
  arc A2628 (-355.7302, 49.25) -> (-355.2311, 49.5618) centre (-355.73, 49.805) ccw
  arc A2629 (-355.2311, 49.5618) -> (-355.1385, 49.8696) centre (-356.13, 50) ccw
  arc A2630 (-354.9898, 50) -> (-355.1385, 49.8696) centre (-354.9898, 49.85) ccw
  line L349 (-354.9898, 50) -> (-354.4705, 50)
  arc A2631 (-354.3218, 49.8696) -> (-354.4705, 50) centre (-354.4705, 49.85) ccw
  arc A2632 (-354.3218, 49.8696) -> (-354.2292, 49.5618) centre (-353.3304, 50) ccw
  arc A2633 (-354.2292, 49.5618) -> (-353.7302, 49.25) centre (-353.7304, 49.805) ccw
  arc A2634 (-353.7302, 49.25) -> (-353.2311, 49.5618) centre (-353.73, 49.805) ccw
  arc A2635 (-353.2311, 49.5618) -> (-353.1385, 49.8696) centre (-354.13, 50) ccw
  arc A2636 (-352.9898, 50) -> (-353.1385, 49.8696) centre (-352.9898, 49.85) ccw
  line L350 (-352.9898, 50) -> (-352.4705, 50)
  arc A2637 (-352.3218, 49.8696) -> (-352.4705, 50) centre (-352.4705, 49.85) ccw
  arc A2638 (-352.3218, 49.8696) -> (-352.2292, 49.5618) centre (-351.3304, 50) ccw
  arc A2639 (-352.2292, 49.5618) -> (-351.7302, 49.25) centre (-351.7304, 49.805) ccw
  arc A2640 (-351.7302, 49.25) -> (-351.2311, 49.5618) centre (-351.73, 49.805) ccw
  arc A2641 (-351.2311, 49.5618) -> (-351.1385, 49.8696) centre (-352.13, 50) ccw
  arc A2642 (-350.9898, 50) -> (-351.1385, 49.8696) centre (-350.9898, 49.85) ccw
  line L351 (-350.9898, 50) -> (-350.4705, 50)
  arc A2643 (-350.3218, 49.8696) -> (-350.4705, 50) centre (-350.4705, 49.85) ccw
  arc A2644 (-350.3218, 49.8696) -> (-350.2292, 49.5618) centre (-349.3304, 50) ccw
  arc A2645 (-350.2292, 49.5618) -> (-349.7302, 49.25) centre (-349.7304, 49.805) ccw
  arc A2646 (-349.7302, 49.25) -> (-349.2311, 49.5618) centre (-349.73, 49.805) ccw
  arc A2647 (-349.2311, 49.5618) -> (-349.1385, 49.8696) centre (-350.13, 50) ccw
  arc A2648 (-348.9898, 50) -> (-349.1385, 49.8696) centre (-348.9898, 49.85) ccw
  line L352 (-348.9898, 50) -> (-348.4705, 50)
  arc A2649 (-348.3218, 49.8696) -> (-348.4705, 50) centre (-348.4705, 49.85) ccw
  arc A2650 (-348.3218, 49.8696) -> (-348.2292, 49.5618) centre (-347.3304, 50) ccw
  arc A2651 (-348.2292, 49.5618) -> (-347.7302, 49.25) centre (-347.7304, 49.805) ccw
  arc A2652 (-347.7302, 49.25) -> (-347.2311, 49.5618) centre (-347.73, 49.805) ccw
  arc A2653 (-347.2311, 49.5618) -> (-347.1385, 49.8696) centre (-348.13, 50) ccw
  arc A2654 (-346.9898, 50) -> (-347.1385, 49.8696) centre (-346.9898, 49.85) ccw
  line L353 (-346.9898, 50) -> (-346.4705, 50)
  arc A2655 (-346.3218, 49.8696) -> (-346.4705, 50) centre (-346.4705, 49.85) ccw
  arc A2656 (-346.3218, 49.8696) -> (-346.2292, 49.5618) centre (-345.3304, 50) ccw
  arc A2657 (-346.2292, 49.5618) -> (-345.7302, 49.25) centre (-345.7304, 49.805) ccw
  arc A2658 (-345.7302, 49.25) -> (-345.2311, 49.5618) centre (-345.73, 49.805) ccw
  arc A2659 (-345.2311, 49.5618) -> (-345.1385, 49.8696) centre (-346.13, 50) ccw
  arc A2660 (-344.9898, 50) -> (-345.1385, 49.8696) centre (-344.9898, 49.85) ccw
  line L354 (-344.9898, 50) -> (-344.4705, 50)
  arc A2661 (-344.3218, 49.8696) -> (-344.4705, 50) centre (-344.4705, 49.85) ccw
  arc A2662 (-344.3218, 49.8696) -> (-344.2292, 49.5618) centre (-343.3304, 50) ccw
  arc A2663 (-344.2292, 49.5618) -> (-343.7302, 49.25) centre (-343.7304, 49.805) ccw
  arc A2664 (-343.7302, 49.25) -> (-343.2311, 49.5618) centre (-343.73, 49.805) ccw
  arc A2665 (-343.2311, 49.5618) -> (-343.1385, 49.8696) centre (-344.13, 50) ccw
  arc A2666 (-342.9898, 50) -> (-343.1385, 49.8696) centre (-342.9898, 49.85) ccw
  line L355 (-342.9898, 50) -> (-342.4705, 50)
  arc A2667 (-342.3218, 49.8696) -> (-342.4705, 50) centre (-342.4705, 49.85) ccw
  arc A2668 (-342.3218, 49.8696) -> (-342.2292, 49.5618) centre (-341.3304, 50) ccw
  arc A2669 (-342.2292, 49.5618) -> (-341.7302, 49.25) centre (-341.7304, 49.805) ccw
  arc A2670 (-341.7302, 49.25) -> (-341.2311, 49.5618) centre (-341.73, 49.805) ccw
  arc A2671 (-341.2311, 49.5618) -> (-341.1385, 49.8696) centre (-342.13, 50) ccw
  arc A2672 (-340.9898, 50) -> (-341.1385, 49.8696) centre (-340.9898, 49.85) ccw
  line L356 (-340.9898, 50) -> (-340.4705, 50)
  arc A2673 (-340.3218, 49.8696) -> (-340.4705, 50) centre (-340.4705, 49.85) ccw
  arc A2674 (-340.3218, 49.8696) -> (-340.2292, 49.5618) centre (-339.3304, 50) ccw
  arc A2675 (-340.2292, 49.5618) -> (-339.7302, 49.25) centre (-339.7304, 49.805) ccw
  arc A2676 (-339.7302, 49.25) -> (-339.2311, 49.5618) centre (-339.73, 49.805) ccw
  arc A2677 (-339.2311, 49.5618) -> (-339.1385, 49.8696) centre (-340.13, 50) ccw
  arc A2678 (-338.9898, 50) -> (-339.1385, 49.8696) centre (-338.9898, 49.85) ccw
  line L357 (-338.9898, 50) -> (-338.4705, 50)
  arc A2679 (-338.3218, 49.8696) -> (-338.4705, 50) centre (-338.4705, 49.85) ccw
  arc A2680 (-338.3218, 49.8696) -> (-338.2292, 49.5618) centre (-337.3304, 50) ccw
  arc A2681 (-338.2292, 49.5618) -> (-337.7302, 49.25) centre (-337.7304, 49.805) ccw
  arc A2682 (-337.7302, 49.25) -> (-337.2311, 49.5618) centre (-337.73, 49.805) ccw
  arc A2683 (-337.2311, 49.5618) -> (-337.1385, 49.8696) centre (-338.13, 50) ccw
  arc A2684 (-336.9898, 50) -> (-337.1385, 49.8696) centre (-336.9898, 49.85) ccw
  line L358 (-336.9898, 50) -> (-336.4705, 50)
  arc A2685 (-336.3218, 49.8696) -> (-336.4705, 50) centre (-336.4705, 49.85) ccw
  arc A2686 (-336.3218, 49.8696) -> (-336.2292, 49.5618) centre (-335.3304, 50) ccw
  arc A2687 (-336.2292, 49.5618) -> (-335.7302, 49.25) centre (-335.7304, 49.805) ccw
  arc A2688 (-335.7302, 49.25) -> (-335.2311, 49.5618) centre (-335.73, 49.805) ccw
  arc A2689 (-335.2311, 49.5618) -> (-335.1385, 49.8696) centre (-336.13, 50) ccw
  arc A2690 (-334.9898, 50) -> (-335.1385, 49.8696) centre (-334.9898, 49.85) ccw
  line L359 (-334.9898, 50) -> (-334.4705, 50)
  arc A2691 (-334.3218, 49.8696) -> (-334.4705, 50) centre (-334.4705, 49.85) ccw
  arc A2692 (-334.3218, 49.8696) -> (-334.2292, 49.5618) centre (-333.3304, 50) ccw
  arc A2693 (-334.2292, 49.5618) -> (-333.7302, 49.25) centre (-333.7304, 49.805) ccw
  arc A2694 (-333.7302, 49.25) -> (-333.2311, 49.5618) centre (-333.73, 49.805) ccw
  arc A2695 (-333.2311, 49.5618) -> (-333.1385, 49.8696) centre (-334.13, 50) ccw
  arc A2696 (-332.9898, 50) -> (-333.1385, 49.8696) centre (-332.9898, 49.85) ccw
  line L360 (-332.9898, 50) -> (-332.4705, 50)
  arc A2697 (-332.3218, 49.8696) -> (-332.4705, 50) centre (-332.4705, 49.85) ccw
  arc A2698 (-332.3218, 49.8696) -> (-332.2292, 49.5618) centre (-331.3304, 50) ccw
  arc A2699 (-332.2292, 49.5618) -> (-331.7302, 49.25) centre (-331.7304, 49.805) ccw
  arc A2700 (-331.7302, 49.25) -> (-331.2311, 49.5618) centre (-331.73, 49.805) ccw
  arc A2701 (-331.2311, 49.5618) -> (-331.1385, 49.8696) centre (-332.13, 50) ccw
  arc A2702 (-330.9898, 50) -> (-331.1385, 49.8696) centre (-330.9898, 49.85) ccw
  line L361 (-330.9898, 50) -> (-330.4705, 50)
  arc A2703 (-330.3218, 49.8696) -> (-330.4705, 50) centre (-330.4705, 49.85) ccw
  arc A2704 (-330.3218, 49.8696) -> (-330.2292, 49.5618) centre (-329.3304, 50) ccw
  arc A2705 (-330.2292, 49.5618) -> (-329.7302, 49.25) centre (-329.7304, 49.805) ccw
  arc A2706 (-329.7302, 49.25) -> (-329.2311, 49.5618) centre (-329.73, 49.805) ccw
  arc A2707 (-329.2311, 49.5618) -> (-329.1385, 49.8696) centre (-330.13, 50) ccw
  arc A2708 (-328.9898, 50) -> (-329.1385, 49.8696) centre (-328.9898, 49.85) ccw
  line L362 (-328.9898, 50) -> (-328.4705, 50)
  arc A2709 (-328.3218, 49.8696) -> (-328.4705, 50) centre (-328.4705, 49.85) ccw
  arc A2710 (-328.3218, 49.8696) -> (-328.2292, 49.5618) centre (-327.3304, 50) ccw
  arc A2711 (-328.2292, 49.5618) -> (-327.7302, 49.25) centre (-327.7304, 49.805) ccw
  arc A2712 (-321.2311, 49.5618) -> (-321.1385, 49.8696) centre (-322.13, 50) ccw
  arc A2713 (-320.9898, 50) -> (-321.1385, 49.8696) centre (-320.9898, 49.85) ccw
  line L363 (-320.9898, 50) -> (-320.4705, 50)
  arc A2714 (-320.3218, 49.8696) -> (-320.4705, 50) centre (-320.4705, 49.85) ccw
  arc A2715 (-320.3218, 49.8696) -> (-320.2292, 49.5618) centre (-319.3304, 50) ccw
  arc A2716 (-320.2292, 49.5618) -> (-319.7302, 49.25) centre (-319.7304, 49.805) ccw
  arc A2717 (-319.7302, 49.25) -> (-319.2311, 49.5618) centre (-319.73, 49.805) ccw
  arc A2718 (-319.2311, 49.5618) -> (-319.1385, 49.8696) centre (-320.13, 50) ccw
  arc A2719 (-318.9898, 50) -> (-319.1385, 49.8696) centre (-318.9898, 49.85) ccw
  line L364 (-318.9898, 50) -> (-318.4705, 50)
  arc A2720 (-318.3218, 49.8696) -> (-318.4705, 50) centre (-318.4705, 49.85) ccw
  arc A2721 (-318.3218, 49.8696) -> (-318.2292, 49.5618) centre (-317.3304, 50) ccw
  arc A2722 (-318.2292, 49.5618) -> (-317.7302, 49.25) centre (-317.7304, 49.805) ccw
  arc A2723 (-317.7302, 49.25) -> (-317.2311, 49.5618) centre (-317.73, 49.805) ccw
  arc A2724 (-317.2311, 49.5618) -> (-317.1385, 49.8696) centre (-318.13, 50) ccw
  arc A2725 (-316.9898, 50) -> (-317.1385, 49.8696) centre (-316.9898, 49.85) ccw
  line L365 (-316.9898, 50) -> (-316.4705, 50)
  arc A2726 (-316.3218, 49.8696) -> (-316.4705, 50) centre (-316.4705, 49.85) ccw
  arc A2727 (-316.3218, 49.8696) -> (-316.2292, 49.5618) centre (-315.3304, 50) ccw
  arc A2728 (-316.2292, 49.5618) -> (-315.7302, 49.25) centre (-315.7304, 49.805) ccw
  arc A2729 (-315.7302, 49.25) -> (-315.2311, 49.5618) centre (-315.73, 49.805) ccw
  arc A2730 (-315.2311, 49.5618) -> (-315.1385, 49.8696) centre (-316.13, 50) ccw
  arc A2731 (-314.9898, 50) -> (-315.1385, 49.8696) centre (-314.9898, 49.85) ccw
  line L366 (-314.9898, 50) -> (-314.4705, 50)
  arc A2732 (-314.3218, 49.8696) -> (-314.4705, 50) centre (-314.4705, 49.85) ccw
  arc A2733 (-314.3218, 49.8696) -> (-314.2292, 49.5618) centre (-313.3304, 50) ccw
  arc A2734 (-314.2292, 49.5618) -> (-313.7302, 49.25) centre (-313.7304, 49.805) ccw
  arc A2735 (-313.7302, 49.25) -> (-313.2311, 49.5618) centre (-313.73, 49.805) ccw
  arc A2736 (-313.2311, 49.5618) -> (-313.1385, 49.8696) centre (-314.13, 50) ccw
  arc A2737 (-312.9898, 50) -> (-313.1385, 49.8696) centre (-312.9898, 49.85) ccw
  line L367 (-312.9898, 50) -> (-312.4705, 50)
  arc A2738 (-312.3218, 49.8696) -> (-312.4705, 50) centre (-312.4705, 49.85) ccw
  arc A2739 (-312.3218, 49.8696) -> (-312.2292, 49.5618) centre (-311.3304, 50) ccw
  arc A2740 (-312.2292, 49.5618) -> (-311.7302, 49.25) centre (-311.7304, 49.805) ccw
  arc A2741 (-311.7302, 49.25) -> (-311.2311, 49.5618) centre (-311.73, 49.805) ccw
  arc A2742 (-311.2311, 49.5618) -> (-311.1385, 49.8696) centre (-312.13, 50) ccw
  arc A2743 (-310.9898, 50) -> (-311.1385, 49.8696) centre (-310.9898, 49.85) ccw
  line L368 (-310.9898, 50) -> (-310.4705, 50)
  arc A2744 (-310.3218, 49.8696) -> (-310.4705, 50) centre (-310.4705, 49.85) ccw
  arc A2745 (-310.3218, 49.8696) -> (-310.2292, 49.5618) centre (-309.3304, 50) ccw
  arc A2746 (-310.2292, 49.5618) -> (-309.7302, 49.25) centre (-309.7304, 49.805) ccw
  arc A2747 (-309.7302, 49.25) -> (-309.2311, 49.5618) centre (-309.73, 49.805) ccw
  arc A2748 (-309.2311, 49.5618) -> (-309.1385, 49.8696) centre (-310.13, 50) ccw
  arc A2749 (-308.9898, 50) -> (-309.1385, 49.8696) centre (-308.9898, 49.85) ccw
  line L369 (-308.9898, 50) -> (-308.4705, 50)
  arc A2750 (-308.3218, 49.8696) -> (-308.4705, 50) centre (-308.4705, 49.85) ccw
  arc A2751 (-308.3218, 49.8696) -> (-308.2292, 49.5618) centre (-307.3304, 50) ccw
  arc A2752 (-308.2292, 49.5618) -> (-307.7302, 49.25) centre (-307.7304, 49.805) ccw
  arc A2753 (-307.7302, 49.25) -> (-307.2311, 49.5618) centre (-307.73, 49.805) ccw
  arc A2754 (-307.2311, 49.5618) -> (-307.1385, 49.8696) centre (-308.13, 50) ccw
  arc A2755 (-306.9898, 50) -> (-307.1385, 49.8696) centre (-306.9898, 49.85) ccw
  line L370 (-306.9898, 50) -> (-306.4705, 50)
  arc A2756 (-306.3218, 49.8696) -> (-306.4705, 50) centre (-306.4705, 49.85) ccw
  arc A2757 (-306.3218, 49.8696) -> (-306.2292, 49.5618) centre (-305.3304, 50) ccw
  arc A2758 (-306.2292, 49.5618) -> (-305.7302, 49.25) centre (-305.7304, 49.805) ccw
  arc A2759 (-305.7302, 49.25) -> (-305.2311, 49.5618) centre (-305.73, 49.805) ccw
  arc A2760 (-305.2311, 49.5618) -> (-305.1385, 49.8696) centre (-306.13, 50) ccw
  arc A2761 (-304.9898, 50) -> (-305.1385, 49.8696) centre (-304.9898, 49.85) ccw
  line L371 (-304.9898, 50) -> (-304.4705, 50)
  arc A2762 (-304.3218, 49.8696) -> (-304.4705, 50) centre (-304.4705, 49.85) ccw
  arc A2763 (-304.3218, 49.8696) -> (-304.2292, 49.5618) centre (-303.3304, 50) ccw
  arc A2764 (-304.2292, 49.5618) -> (-303.7302, 49.25) centre (-303.7304, 49.805) ccw
  arc A2765 (-303.7302, 49.25) -> (-303.2311, 49.5618) centre (-303.73, 49.805) ccw
  arc A2766 (-303.2311, 49.5618) -> (-303.1385, 49.8696) centre (-304.13, 50) ccw
  arc A2767 (-302.9898, 50) -> (-303.1385, 49.8696) centre (-302.9898, 49.85) ccw
  line L372 (-302.9898, 50) -> (-302.4705, 50)
  arc A2768 (-302.3218, 49.8696) -> (-302.4705, 50) centre (-302.4705, 49.85) ccw
  arc A2769 (-302.3218, 49.8696) -> (-302.2292, 49.5618) centre (-301.3304, 50) ccw
  arc A2770 (-302.2292, 49.5618) -> (-301.7302, 49.25) centre (-301.7304, 49.805) ccw
  arc A2771 (-301.7302, 49.25) -> (-301.2311, 49.5618) centre (-301.73, 49.805) ccw
  arc A2772 (-301.2311, 49.5618) -> (-301.1385, 49.8696) centre (-302.13, 50) ccw
  arc A2773 (-300.9898, 50) -> (-301.1385, 49.8696) centre (-300.9898, 49.85) ccw
  line L373 (-300.9898, 50) -> (-300.4705, 50)
  arc A2774 (-300.3218, 49.8696) -> (-300.4705, 50) centre (-300.4705, 49.85) ccw
  arc A2775 (-300.3218, 49.8696) -> (-300.2292, 49.5618) centre (-299.3304, 50) ccw
  arc A2776 (-300.2292, 49.5618) -> (-299.7302, 49.25) centre (-299.7304, 49.805) ccw
  arc A2777 (-299.7302, 49.25) -> (-299.2311, 49.5618) centre (-299.73, 49.805) ccw
  arc A2778 (-299.2311, 49.5618) -> (-299.1385, 49.8696) centre (-300.13, 50) ccw
  arc A2779 (-298.9898, 50) -> (-299.1385, 49.8696) centre (-298.9898, 49.85) ccw
  line L374 (-298.9898, 50) -> (-298.4705, 50)
  arc A2780 (-298.3218, 49.8696) -> (-298.4705, 50) centre (-298.4705, 49.85) ccw
  arc A2781 (-298.3218, 49.8696) -> (-298.2292, 49.5618) centre (-297.3304, 50) ccw
  arc A2782 (-298.2292, 49.5618) -> (-297.7302, 49.25) centre (-297.7304, 49.805) ccw
  arc A2783 (-297.7302, 49.25) -> (-297.2311, 49.5618) centre (-297.73, 49.805) ccw
  arc A2784 (-297.2311, 49.5618) -> (-297.1385, 49.8696) centre (-298.13, 50) ccw
  arc A2785 (-296.9898, 50) -> (-297.1385, 49.8696) centre (-296.9898, 49.85) ccw
  line L375 (-296.9898, 50) -> (-296.4705, 50)
  arc A2786 (-296.3218, 49.8696) -> (-296.4705, 50) centre (-296.4705, 49.85) ccw
  arc A2787 (-296.3218, 49.8696) -> (-296.2292, 49.5618) centre (-295.3304, 50) ccw
  arc A2788 (-296.2292, 49.5618) -> (-295.7302, 49.25) centre (-295.7304, 49.805) ccw
  arc A2789 (-295.7302, 49.25) -> (-295.2311, 49.5618) centre (-295.73, 49.805) ccw
  arc A2790 (-295.2311, 49.5618) -> (-295.1385, 49.8696) centre (-296.13, 50) ccw
  arc A2791 (-294.9898, 50) -> (-295.1385, 49.8696) centre (-294.9898, 49.85) ccw
  line L376 (-294.9898, 50) -> (-294.4705, 50)
  arc A2792 (-294.3218, 49.8696) -> (-294.4705, 50) centre (-294.4705, 49.85) ccw
  arc A2793 (-294.3218, 49.8696) -> (-294.2292, 49.5618) centre (-293.3304, 50) ccw
  arc A2794 (-294.2292, 49.5618) -> (-293.7302, 49.25) centre (-293.7304, 49.805) ccw
  arc A2795 (-293.7302, 49.25) -> (-293.2311, 49.5618) centre (-293.73, 49.805) ccw
  arc A2796 (-293.2311, 49.5618) -> (-293.1385, 49.8696) centre (-294.13, 50) ccw
  arc A2797 (-292.9898, 50) -> (-293.1385, 49.8696) centre (-292.9898, 49.85) ccw
  line L377 (-292.9898, 50) -> (-292.4705, 50)
  arc A2798 (-292.3218, 49.8696) -> (-292.4705, 50) centre (-292.4705, 49.85) ccw
  arc A2799 (-292.3218, 49.8696) -> (-292.2292, 49.5618) centre (-291.3304, 50) ccw
  arc A2800 (-292.2292, 49.5618) -> (-291.7302, 49.25) centre (-291.7304, 49.805) ccw
  arc A2801 (-291.7302, 49.25) -> (-291.2311, 49.5618) centre (-291.73, 49.805) ccw
  arc A2802 (-291.2311, 49.5618) -> (-291.1385, 49.8696) centre (-292.13, 50) ccw
  arc A2803 (-290.9898, 50) -> (-291.1385, 49.8696) centre (-290.9898, 49.85) ccw
  line L378 (-290.9898, 50) -> (-290.4705, 50)
  arc A2804 (-290.3218, 49.8696) -> (-290.4705, 50) centre (-290.4705, 49.85) ccw
  arc A2805 (-290.3218, 49.8696) -> (-290.2292, 49.5618) centre (-289.3304, 50) ccw
  arc A2806 (-290.2292, 49.5618) -> (-289.7302, 49.25) centre (-289.7304, 49.805) ccw
  arc A2807 (-289.7302, 49.25) -> (-289.2311, 49.5618) centre (-289.73, 49.805) ccw
  arc A2808 (-289.2311, 49.5618) -> (-289.1385, 49.8696) centre (-290.13, 50) ccw
  arc A2809 (-288.9898, 50) -> (-289.1385, 49.8696) centre (-288.9898, 49.85) ccw
  line L379 (-288.9898, 50) -> (-288.4705, 50)
  arc A2810 (-288.3218, 49.8696) -> (-288.4705, 50) centre (-288.4705, 49.85) ccw
  arc A2811 (-288.3218, 49.8696) -> (-288.2292, 49.5618) centre (-287.3304, 50) ccw
  arc A2812 (-288.2292, 49.5618) -> (-287.7302, 49.25) centre (-287.7304, 49.805) ccw
  arc A2813 (-287.7302, 49.25) -> (-287.2311, 49.5618) centre (-287.73, 49.805) ccw
  arc A2814 (-287.2311, 49.5618) -> (-287.1385, 49.8696) centre (-288.13, 50) ccw
  arc A2815 (-286.9898, 50) -> (-287.1385, 49.8696) centre (-286.9898, 49.85) ccw
  line L380 (-286.9898, 50) -> (-286.4705, 50)
  arc A2816 (-286.3218, 49.8696) -> (-286.4705, 50) centre (-286.4705, 49.85) ccw
  arc A2817 (-286.3218, 49.8696) -> (-286.2292, 49.5618) centre (-285.3304, 50) ccw
  arc A2818 (-286.2292, 49.5618) -> (-285.7302, 49.25) centre (-285.7304, 49.805) ccw
  arc A2819 (-285.7302, 49.25) -> (-285.2311, 49.5618) centre (-285.73, 49.805) ccw
  arc A2820 (-285.2311, 49.5618) -> (-285.1385, 49.8696) centre (-286.13, 50) ccw